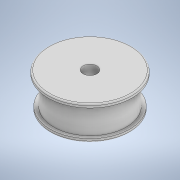
# Autodesk Inventor part: rail wheel
Saved by Autodesk Inventor 2022 (Build 260153000, 153)
## iProperties
Created: 2021-11-07
Part Number: rail wheel
Material: Generic
Document SubType Name: Modeling
Designer: kibandi
Density: 1 g/cm^3
Appearance: Default
Author: kibandi
Autodesk Inventor part; units mm, degrees
ref_plane "YZ Plane" through (0, 0, 0) normal (1, 0, 0) x (0, 1, 0)
ref_plane "XZ Plane" through (0, 0, 0) normal (0, 1, 0) x (-1, 0, 0)
ref_plane "XY Plane" through (0, 0, 0) normal (0, 0, 1) x (1, 0, 0)
sketch "Sketch1" plane through (0, 0, 0) normal (0, 0, 1) x (1, 0, 0)
  line L0 (0, 0) -> (0, 50)
  line L1 (-10, 50) -> (-58, 50)
  line L2 (-60, 48) -> (-60, 45)
  line L3 (-60, 45) -> (-52, 45)
  line L4 (-52, 45) -> (-52, 5)
  line L5 (-52, 5) -> (-57, 5)
  line L6 (-57, 5) -> (-57, 2)
  line L7 (-55, 0) -> (-10, 0)
  line L8 (-10, 0) -> (-10, 50)
  arc A0 (-58, 50) -> (-60, 48) centre (-58, 48) ccw
  arc A1 (-57, 2) -> (-55, 0) centre (-55, 2) ccw
  point P0 (-60, 50)
  point P1 (-57, 0)
  dimension "d0" = 50
  dimension "d1" = 10
  dimension "d2" = 50
  dimension "d3" = 5
  dimension "d4" = 8
  dimension "d5" = 40
  dimension "d6" = 5
  dimension "d7" = 47
  dimension "d8" = 2
  constraints: 18 end point, 5 perpendicular, 4 point on circle, 4 point on line, 4 tangent, 2 centre point, 1 equal radius, 1 horizontal, 1 vertical
  measures "d0" distance of L0.start L0.end
  measures "d1" distance of L0.end L1.start
  measures "d2" distance of L1.start point (-60, 50)
  measures "d3" distance of point (-60, 50) L2.end
  measures "d4" distance of L2.end L3.end
  measures "d5" distance of L3.end L4.end
  measures "d6" distance of L4.end L5.end
  measures "d7" distance of point (-57, 0) L7.end
  measures "d8" radius of A0
revolve "Revolution1" add sketch "Sketch1" angle 360 about axis through (0, 0, 0) along (0, 1, 0)
body "Solid1"
